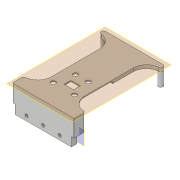
# Autodesk Inventor part: Mount_new
Saved by Autodesk Inventor 2019 (Build 230136000, 136)
## iProperties
Created: 2021-06-04
Part Number: Mount_new
Material: Generic
Document SubType Name: Sheet Metal
Designer: wanghaoran
Density: 1 g/cm^3
Sheet Metal Rule: Default
Appearance: Default
Author: wanghaoran
Autodesk Inventor part; units mm, degrees
ref_plane "YZ Plane" through (0, 0, 0) normal (1, 0, 0) x (0, 1, 0)
ref_plane "XZ Plane" through (0, 0, 0) normal (0, 1, 0) x (-1, 0, 0)
ref_plane "XY Plane" through (0, 0, 0) normal (0, 0, 1) x (1, 0, 0)
ref_plane "Work Plane1" through (-26.3558, 20.5023, 45.2893) normal (0, 1, 0) x (-1, 0, 0)
sketch "Sketch1" plane through (-26.3558, 20.5023, 45.2893) normal (0, 1, 0) x (-1, 0, 0)
  line L0 (21.35, 36.9014) -> (-69.35, 36.9014) projected
  arc A0 (-67.1927, -92.9954) -> (-49, -73.0268) centre (-69.0003, -73.0769) ccw
  line L1 (-66.85, -99.9786) -> (18.85, -99.9786) projected
  line L2 (1, -73.0771) -> (1, 0) projected
  line L3 (22.35, 23.4014) -> (22.35, 35.9015) projected
  line L4 (22.35, 35.9015) -> (21.35, 36.9014) projected
  line L5 (-69.35, 36.9014) -> (-70.35, 35.9015) projected
  line L6 (-70.35, 35.9015) -> (-70.35, 23.4014) projected
  arc A1 (19.0233, 19.8966) -> (22.35, 23.4014) centre (18.8404, 23.4014) ccw
  arc A2 (19.0233, 19.8966) -> (1, 0) centre (21, -0.0055) ccw
  arc A3 (18.85, -99.9786) -> (19.1351, -92.9903) centre (18.85, -96.4786) ccw
  arc A4 (1, -73.0771) -> (19.1351, -92.9903) centre (21.0003, -73.0771) ccw
  arc A5 (-70.35, 23.4014) -> (-66.9693, 19.8966) centre (-66.85, 23.3946) ccw
  line L7 (-49, 0) -> (-49, -73.0771) projected
  arc A6 (-49, 0) -> (-66.9693, 19.8966) centre (-69, 0) ccw
  arc A7 (-67.1927, -92.9954) -> (-66.85, -99.9786) centre (-66.85, -96.4786) ccw
  circle A8 centre (-7.9999, 5.9015) radius 3.5001 projected
  circle A9 centre (-14.5002, -21.099) radius 3.4996 projected
  circle A10 centre (-40.0001, 5.9014) radius 3.4999 projected
  circle A11 centre (-33.4996, -21.0984) radius 3.5005 projected
  point P0 (-26.3558, -45.2893)
  dimension "d0" = 20
  dimension "d1" = 3.5
  dimension "d2" = 20
  constraints: 16 point on circle, 8 centre point, 3 tangent, 1 point on line
  measures "d0" radius of A2
  measures "d1" radius of A5
  measures "d2" radius of A6
extrude "Extrusion1" add sketch "Sketch1" against normal blind 5
sketch "Sketch2" plane through (-26.3558, 15.5023, 45.2893) normal (0, -1, 0) x (1, 0, 0)
  line L0 (-22.35, 35.9015) -> (-22.35, 23.4014) projected
  arc A0 (-22.35, 23.4014) -> (-19.0233, 19.8966) centre (-18.8404, 23.4014) ccw projected
  line L1 (69.35, 36.9014) -> (-21.35, 36.9014) projected
  line L2 (-21.35, 36.9014) -> (-22.35, 35.9015) projected
  line L3 (70.35, 35.9015) -> (69.35, 36.9014) projected
  line L4 (70.35, 23.4014) -> (70.35, 35.9015) projected
  arc A1 (66.9693, 19.8966) -> (70.35, 23.4014) centre (66.85, 23.3946) ccw projected
  arc A2 (66.9693, 19.8966) -> (49, 0) centre (69, 0) ccw projected
  line L5 (-19.0233, 19.8966) -> (66.9693, 19.8966)
  circle A3 centre (-18.85, 23.4014) radius 1.45 projected
  circle A4 centre (66.8502, 23.4017) radius 1.4503 projected
  circle A5 centre (-18.85, -96.4785) radius 3.5 projected
  circle A6 centre (-18.85, -96.4786) radius 1.45 projected
  circle A7 centre (66.85, -96.4785) radius 3.5001 projected
  circle A8 centre (66.8502, -96.4783) radius 1.4503 projected
  circle A9 centre (-18.85, 23.4014) radius 1.5
  circle A10 centre (66.8502, 23.4017) radius 1.4003
  circle A11 centre (66.8502, -96.4783) radius 1.4003
  circle A12 centre (-18.85, -96.4786) radius 1.4
  point P0 (26.3558, -45.2893)
  dimension "d43" = 0.05
  dimension "d44" = 0.05
  dimension "d45" = 0.05
  dimension "d46" = 0.05
  constraints: 4 centre point, 2 end point, 1 horizontal
  measures "d43" radial gap between concentric circles of A3 A9
  measures "d44" radial gap between concentric circles of A4 A10
  measures "d45" radial gap between concentric circles of A8 A11
  measures "d46" radial gap between concentric circles of A6 A12
ref_plane "Work Plane2" through (-26.3558, -4.9977, 45.2893) normal (0, -1, 0) x (1, 0, 0)
sketch "Sketch3" plane through (-26.3558, -4.9977, 45.2893) normal (0, -1, 0) x (1, 0, 0)
  line L0 (-21.35, 36.9014) -> (69.35, 36.9014) projected
  line L1 (-18.35, 36.9014) -> (66.35, 36.9014)
  line L2 (66.35, 36.9014) -> (66.35, 28.9014)
  line L3 (66.35, 28.9014) -> (-18.35, 28.9014)
  line L4 (-18.35, 28.9014) -> (-18.35, 36.9014)
  line L5 (-22.35, 35.9015) -> (-22.35, 23.4014) projected
  point P0 (26.3558, -45.2893)
  dimension "d9" = 84.7
  dimension "d10" = 8
  dimension "d11" = 4
  constraints: 8 end point, 2 parallel, 1 horizontal, 1 perpendicular, 1 point on line
  measures "d9" distance of L2.end L3.end
  measures "d10" distance of L1.end L2.end
  measures "d11" distance between parallel lines of L5 L4
extrude "Extrusion4" add sketch "Sketch3" along normal blind 13.5
ref_plane "Work Plane3" through (39.9942, -4.9977, 74.1907) normal (0, 0, -1) x (-1, 0, 0)
sketch "Sketch4" plane through (39.9942, -4.9977, 74.1907) normal (0, 0, -1) x (-1, 0, 0)
  circle A0 centre (67.3499, -6.5) radius 5.2499 projected
  circle A1 centre (42.3495, -6.5001) radius 5.2495 projected
  line L0 (0, 0) -> (0, -13.5) projected
  line L1 (84.7, -13.5) -> (0, -13.5) projected
  line L2 (84.7, 0) -> (84.7, -13.5) projected
  circle A2 centre (17.3499, -6.5002) radius 5.2498 projected
  line L3 (0, 0) -> (84.7, 0) projected
  point P0 (39.9942, 4.9977)
  point P1 (17.5275, -7.0805)
hole "Hole2" at (-27.3557, -11.4977, 74.1907) at (-2.3553, -11.4978, 74.1907) at (22.4667, -12.0781, 74.1907) direction (0, 0, 1) diameter 4.6 end through all counterbore diameter 10.5 counterbore depth 5
sketch "Sketch5" plane through (-26.3558, 15.5023, 45.2893) normal (0, -1, 0) x (1, 0, 0)
  line L0 (-1, -42.0986) -> (49, -42.0986)
  line L1 (49, -42.0986) -> (49, 11.9014)
  line L2 (49, 11.9014) -> (-1, 11.9014)
  line L3 (-1, 11.9014) -> (-1, -42.0986)
  circle A0 centre (40.0001, 5.9014) radius 3.4999 projected
  arc A1 (66.9693, 19.8966) -> (49, 0) centre (69, 0) ccw projected
  line L4 (49, -42.0986) -> (53.7175, -42.0986)
  line L5 (53.7175, -42.0986) -> (53.7175, 11.9014)
  line L6 (53.7175, 11.9014) -> (49, 11.9014)
  line L7 (49, 11.9014) -> (49, -42.0986)
  arc A2 (-1, 0) -> (-19.0233, 19.8966) centre (-21, -0.0055) ccw projected
  arc A3 (-1, 0) -> (-19.0233, 19.8966) centre (-21, -0.0055) ccw projected
  line L8 (-1, -42.0986) -> (-4.9306, -42.0986)
  line L9 (-4.9306, -42.0986) -> (-4.9306, 11.9014)
  line L10 (-4.9306, 11.9014) -> (-1, 11.9014)
  line L11 (-1, 11.9014) -> (-1, -42.0986)
  line L12 (49, 11.9014) -> (-1, 11.9014)
  line L13 (-1, 11.9014) -> (-1, -42.0986)
  line L14 (-1, -42.0986) -> (49, -42.0986)
  line L15 (49, -42.0986) -> (49, 11.9014)
  point P0 (26.3558, -45.2893)
  dimension "d28" = 50
  dimension "d29" = 54
  dimension "d30" = 6
  dimension "d37" = 54
  constraints: 32 end point, 8 parallel, 4 horizontal, 4 perpendicular, 1 point on circle
  measures "d28" distance of L2.end L1.end
  measures "d29" distance of L1.start L1.end
  measures "d30" distance from line of A0.centre L2
  measures "d37" distance of L4.end L5.end
extrude "Extrusion5" cut sketch "Sketch5" against normal blind 3.5
sketch "Sketch6" plane through (-26.3558, 19.0023, 45.2893) normal (0, -1, 0) x (1, 0, 0)
  line L0 (32.4999, -0.0986) -> (18.4999, -0.0986)
  line L1 (18.4999, -0.0986) -> (18.4999, -10.0986)
  line L2 (18.4999, -10.0986) -> (32.4999, -10.0986)
  line L3 (32.4999, -10.0986) -> (32.4999, -0.0986)
  line L4 (-1, 11.9014) -> (49, 11.9014) projected
  circle A0 centre (7.9999, 5.9015) radius 3.5001 projected
  point P0 (26.3558, -45.2893)
  point P1 (-5.7221, 12.9014)
  point P2 (53.7175, 12.9014)
  dimension "d33" = 14
  dimension "d34" = 10
  dimension "d36" = 22
  dimension "d40" = 10.5
  constraints: 8 end point, 2 parallel, 1 horizontal, 1 perpendicular, 1 other
  measures "d33" distance of L2.end L1.end
  measures "d34" distance of L1.end L0.end
  measures "d40" distance from line of A0.centre L1
extrude "Extrusion6" cut sketch "Sketch6" against normal through all contours L3 L2 L1 L0
extrude "Extrusion7" add sketch "Sketch2" along normal blind 20.5 contours L2 L1 L3 L4 A1 L5 A0 L0 | A4 | A5 | A6 | A7 | A8 | A9
sketch "Sketch7" plane through (-26.3558, -4.9977, 45.2893) normal (0, -1, 0) x (1, 0, 0)
  line L0 (66.9693, 19.8966) -> (-19.0233, 19.8966) projected
  line L1 (62.9499, 19.8966) -> (-15.0501, 19.8966)
  line L2 (-15.0501, 19.8966) -> (-15.0501, 25.8966)
  line L3 (-15.0501, 25.8966) -> (62.9499, 25.8966)
  line L4 (62.9499, 25.8966) -> (62.9499, 19.8966)
  circle A0 centre (66.8502, 23.4017) radius 1.4003 projected
  point P0 (26.3558, -45.2893)
  dimension "d49" = 78
  dimension "d50" = 6
  dimension "d51" = 2.5
  constraints: 8 end point, 2 parallel, 1 horizontal, 1 perpendicular, 1 point on line
  measures "d49" distance of L2.end L3.end
  measures "d50" distance of L1.end L2.end
  measures "d51" distance edge to line of A0 L4
extrude "Extrusion8" cut sketch "Sketch7" against normal blind 13 contours L0 L2 L3 L4
equation "\"d26\" = Thickness"
equation "\"BendRadius\" = Thickness"
equation "\"BendReliefWidth\" = Thickness"
equation "\"BendReliefDepth\" = 0.5 * Thickness"
equation "\"CornerReliefSize\" = 4 * Thickness"
equation "\"MinimumRemnant\" = 2 * Thickness"
equation "\"TransitionRadius\" = BendRadius"
equation "\"JacobiRadiusSize\" = Thickness"
equation "\"GapSize\" = Thickness"
equation "\"Thickness\" = 0.5"
body "Solid1"
